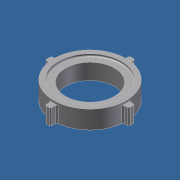
# Autodesk Inventor part: hfc12_panel_tight
Saved by Autodesk Inventor 2012 SP1 (Build 160190100, 190)
## iProperties
Category: PARTsolutions
Created: 2012-06-06
Part Number: hfc12_panel_tight
Catalog Web Link: www.cadenas.de
Description: hfc12_panel_tight - hfc12_panel_tight
Document SubType Name: Modeling
Designer: PARTsolutions
Material: Default
Mass: 6.53088 g
Surface Area: 36.8366 cm^2
Volume: 6.53088 cm^3
Density: 1 g/cm^3
NB: hfc12_panel_tight
NN: hfc12_panel_tight
NT: hfc12_panel_tight
NBSYN: $PN.
LINA: hfc12_panel_tight
PN: hfc12_panel_tight
KT: DUMMY
SUPPLIER: Colder
ARTICLENO: hfc12_panel_tightHI
BOMINFO: hfc12_panel_tight
CREATOR: CADENAS GmbH
PSOL_IDENT_0: {\\10.0.0.251\data_v9\23d-libs\colder\single_line\3_8_nom_flow\hfc12_series\bodies\parts\hfc12_panel
PSOL_IDENT_1: _tight.prj},187 {VTYP=3D},{NB=hfc12_panel_tight},{LINA=hfc12_panel_tight},{NN=hfc12_panel_tight},{DA
PSOL_IDENT_2: TE=08.08.2007 07:17:46},{GEOMDATE=08.08.2007 07:00:00},{VERSION=},{LINEID=10},{LINESUBID=-1},{WBVAR=
PSOL_IDENT_3: }  {NB=hfc12_panel_tight},{LINA=hfc12_panel_tight},{KT=DUMMY},{PN=hfc12_panel_tight}
Title: hfc12_panel_tight
Author: Cadenas PARTsolutions
Comments: hfc12_panel_tight
Autodesk Inventor part; units mm, degrees
sketch "Sketch1" plane through (0, 0, 0) normal (0, 1, 0) x (-1, 0, 0)
  line L0 (0, -43.688) -> (0, -44.958)
  line L1 (0, -44.958) -> (-19.812, -44.958)
  line L2 (-19.812, -44.958) -> (-19.812, -43.688)
  line L3 (-19.812, -43.688) -> (0, -43.688)
  line L4 (0, -43.688) -> (0, -44.958)
  constraints: 10 end point
revolve "Revolution1" add sketch "Sketch1" angle 360 about axis through (0, 0, -43.688) along (0, 0, 1)
sketch "Sketch4" plane through (0, 0, -44.958) normal (0, 0, -1) x (-1, 0, 0)
  arc A0 (-22.7886, -0.9184) -> (-22.0266, -1.6804) centre (-22.0266, -0.9184) ccw
  line L0 (-22.0266, -1.6804) -> (-20.4285, -1.6804)
  arc A1 (-19.6719, -2.3519) -> (-20.4285, -1.6804) centre (-20.4285, -2.4424) ccw
  arc A2 (-19.6719, -2.3519) -> (-2.2013, -19.6893) centre (0, 0) ccw
  arc A3 (-1.524, -20.4466) -> (-2.2013, -19.6893) centre (-2.286, -20.4466) ccw
  line L1 (-1.524, -20.4466) -> (-1.524, -22.352)
  arc A4 (-1.524, -22.352) -> (-0.762, -23.114) centre (-0.762, -22.352) ccw
  line L2 (-0.762, -23.114) -> (0.762, -23.114)
  arc A5 (0.762, -23.114) -> (1.524, -22.352) centre (0.762, -22.352) ccw
  line L3 (1.524, -22.352) -> (1.524, -20.4466)
  arc A6 (2.2013, -19.6893) -> (1.524, -20.4466) centre (2.286, -20.4466) ccw
  arc A7 (2.2013, -19.6893) -> (19.6719, -2.3519) centre (0, 0) ccw
  arc A8 (20.4285, -1.6804) -> (19.6719, -2.3519) centre (20.4285, -2.4424) ccw
  line L4 (20.4285, -1.6804) -> (22.0266, -1.6804)
  arc A9 (22.0266, -1.6804) -> (22.7886, -0.9184) centre (22.0266, -0.9184) ccw
  line L5 (22.7886, -0.9184) -> (22.7886, 0.9184)
  arc A10 (22.7886, 0.9184) -> (22.0266, 1.6804) centre (22.0266, 0.9184) ccw
  line L6 (22.0266, 1.6804) -> (20.4285, 1.6804)
  arc A11 (19.6719, 2.3519) -> (20.4285, 1.6804) centre (20.4285, 2.4424) ccw
  arc A12 (19.6719, 2.3519) -> (2.2013, 19.6893) centre (0, 0) ccw
  arc A13 (1.524, 20.4466) -> (2.2013, 19.6893) centre (2.286, 20.4466) ccw
  line L7 (1.524, 20.4466) -> (1.524, 22.352)
  arc A14 (1.524, 22.352) -> (0.762, 23.114) centre (0.762, 22.352) ccw
  line L8 (0.762, 23.114) -> (-0.762, 23.114)
  arc A15 (-0.762, 23.114) -> (-1.524, 22.352) centre (-0.762, 22.352) ccw
  line L9 (-1.524, 22.352) -> (-1.524, 20.4466)
  arc A16 (-2.2013, 19.6893) -> (-1.524, 20.4466) centre (-2.286, 20.4466) ccw
  arc A17 (-2.2013, 19.6893) -> (-19.6719, 2.3519) centre (0, 0) ccw
  arc A18 (-20.4285, 1.6804) -> (-19.6719, 2.3519) centre (-20.4285, 2.4424) ccw
  line L10 (-20.4285, 1.6804) -> (-22.0266, 1.6804)
  arc A19 (-22.0266, 1.6804) -> (-22.7886, 0.9184) centre (-22.0266, 0.9184) ccw
  line L11 (-22.7886, 0.9184) -> (-22.7886, -0.9184)
  constraints: 40 point on circle, 24 end point, 20 centre point
extrude "Extrusion1" add sketch "Sketch4" along normal blind 8.636
sketch "Sketch7" plane through (0, 0, 0) normal (0, 1, 0) x (-1, 0, 0)
  line L0 (0, -43.688) -> (0, -53.594)
  line L1 (0, -53.594) -> (-13.3629, -53.594)
  line L2 (-13.3629, -53.594) -> (-13.3629, -44.958)
  line L3 (-13.3629, -44.958) -> (-16.891, -44.958)
  arc A0 (-17.272, -44.577) -> (-16.891, -44.958) centre (-16.891, -44.577) ccw
  line L4 (-17.272, -44.577) -> (-17.272, -43.688)
  line L5 (-17.272, -43.688) -> (0, -43.688)
  line L6 (0, -43.688) -> (0, -53.594)
  constraints: 14 end point, 2 point on circle, 1 centre point
revolve "Revolution2" cut sketch "Sketch7" angle 360 about axis through (0, 0, -43.688) along (0, 0, 1)
ref_plane "0_XY" through (0, 0, 0) normal (0, 0, 1) x (1, 0, 0)
ref_plane "0_YZ" through (0, 0, 0) normal (1, 0, 0) x (0, 1, 0)
ref_plane "0_ZX" through (0, 0, 0) normal (0, 1, 0) x (0, 0, 1)
body "Solid1"
